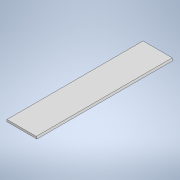
# Autodesk Inventor part: top
Saved by Autodesk Inventor 2021 (Build 250183000, 183)
## iProperties
Created: 2020-07-28
Part Number: top
Material: Generic
Document SubType Name: Modeling
Designer: johna
Density: 1 g/cm^3
Appearance: Default
Author: johna
Autodesk Inventor part; units mm, degrees
ref_plane "YZ Plane" through (0, 0, 0) normal (1, 0, 0) x (0, 1, 0)
ref_plane "XZ Plane" through (0, 0, 0) normal (0, 1, 0) x (-1, 0, 0)
ref_plane "XY Plane" through (0, 0, 0) normal (0, 0, 1) x (1, 0, 0)
sketch "Sketch1" plane through (0, 0, 0) normal (0, 1, 0) x (-1, 0, 0)
  line L0 (3.2185, 25.3311) -> (-34.8815, 25.3311)
  line L1 (-34.8815, 25.3311) -> (-34.8815, -147.3889)
  line L2 (-34.8815, -147.3889) -> (3.2185, -147.3889)
  line L3 (3.2185, -147.3889) -> (3.2185, 25.3311)
  point P0 (0, 0)
  dimension "d0" = 38.1
  dimension "d1" = 172.72
  constraints: 8 end point, 2 parallel, 1 horizontal, 1 perpendicular
  measures "d0" distance of L2.end L1.end
  measures "d1" distance of L1.end L0.end
extrude "Extrusion1" add sketch "Sketch1" along normal blind 2.54
sketch "Sketch2" plane through (-3.2185, 0, 25.3311) normal (0, 0, 1) x (1, 0, 0)
  line L0 (38.1, 0) -> (0, 0) projected
  line L1 (38.1, 0) -> (37.1755, 2.54)
  line L2 (38.1, 2.54) -> (0, 2.54) projected
  line L3 (38.1, 0) -> (38.1, 2.54) projected
  point P0 (3.2185, 0)
  dimension "d4" = 20
  constraints: 2 end point, 1 point on line
  measures "d4" angle of L3 L1
extrude "Extrusion2" cut sketch "Sketch2" against normal blind 172.72
body "Solid1"
